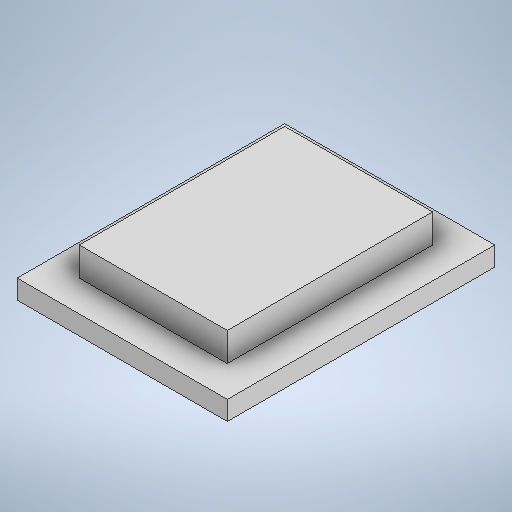
# Autodesk Inventor part: Motor_Fensterdeckel
Saved by Autodesk Inventor 2025 (Build 290162000, 162)
## iProperties
Created: 2026-07-09
Part Number: Motor_Fensterdeckel
Material: Generisch
Document SubType Name: Modeling
Designer: wavid
Mass: 2.23175 g
Surface Area: 23.205 cm^2
Volume: 2.23175 cm^3
Density: 1 g/cm^3
Appearance: Vorgabe
Author: wavid
Autodesk Inventor part; units mm, degrees
ref_plane "YZ Plane" through (0, 0, 0) normal (1, 0, 0) x (0, 1, 0)
ref_plane "XZ Plane" through (0, 0, 0) normal (0, 1, 0) x (-1, 0, 0)
sketch "Skizze1" plane through (0, 0, 0) normal (0, 0, 1) x (1, 0, 0)
  line L0 (-11, -14) -> (11, -14)
  line L1 (11, -14) -> (11, 14)
  line L2 (11, 14) -> (-11, 14)
  line L3 (-11, 14) -> (-11, -14)
  constraints: 8 end point, 2 parallel, 1 horizontal, 1 perpendicular
extrude "Extrusion1" add sketch "Skizze1" along normal blind 2
ref_plane "Arbeitsebene1" through (0, 0, 2) normal (0, 0, 1) x (1, 0, 0)
sketch "Skizze2" plane through (0, 0, 2) normal (0, 0, 1) x (1, 0, 0)
  line L0 (-7.75, -10.75) -> (7.75, -10.75)
  line L1 (7.75, -10.75) -> (7.75, 10.75)
  line L2 (7.75, 10.75) -> (-7.75, 10.75)
  line L3 (-7.75, 10.75) -> (-7.75, -10.75)
  constraints: 8 end point, 2 parallel, 1 horizontal, 1 perpendicular
extrude "Extrusion2" add sketch "Skizze2" along normal blind 3 separate body
